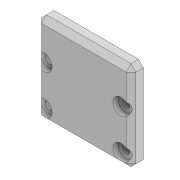
# Autodesk Inventor part: Print_Parts_S2
Saved by Autodesk Inventor 2020.1 (Build 241239000, 239)
## iProperties
Created: 2020-11-09
Part Number: Print_Parts_S2
Material: 一般
Document SubType Name: Modeling
Designer: kenta iguchi
Density: 1 g/cm^3
Appearance: 既定
Author: kenta iguchi
Autodesk Inventor part; units mm, degrees
ref_plane "YZ Plane" through (0, 0, 0) normal (1, 0, 0) x (0, 1, 0)
ref_plane "XZ Plane" through (0, 0, 0) normal (0, 1, 0) x (-1, 0, 0)
ref_plane "XY Plane" through (0, 0, 0) normal (0, 0, 1) x (1, 0, 0)
sketch "スケッチ1" plane through (0, 0, 0) normal (0, 0, 1) x (1, 0, 0)
  line L0 (-19, -18) -> (19, -18)
  line L1 (19, -18) -> (19, 18)
  line L2 (19, 18) -> (-19, 18)
  line L3 (-19, 18) -> (-19, -18)
  line L4 (-19, -18) -> (19, 18) construction
  line L5 (19, -18) -> (-19, 18) construction
  point P0 (0, 0)
  dimension "d0" = 38
  dimension "d1" = 36
  constraints: 12 end point, 2 midpoint, 2 parallel, 1 horizontal, 1 perpendicular
  measures "d0" distance of L2.end L1.end
  measures "d1" distance of L1.end L0.end
extrude "押し出し1" add sketch "スケッチ1" along normal blind 5
chamfer "面取り1" distance 2 angle 45 8 edges at (0, 18, 5) (19, 0, 5) (0, -18, 5) (-19, 0, 5) (19, -18, 2.5) (-19, -18, 2.5) (-19, 18, 2.5) (19, 18, 2.5)
sketch "スケッチ2" plane through (0, 0, 5) normal (0, 0, 1) x (1, 0, 0)
  line L0 (-19, -18) -> (19, -18) projected
  line L1 (19, -18) -> (19, 18) projected
  line L2 (-16, -13) -> (15, -13)
  line L3 (15, -13) -> (15, 3)
  line L4 (15, 3) -> (-16, 3)
  line L5 (-16, 3) -> (-16, -13)
  line L6 (-16, -13) -> (15, 3) construction
  line L7 (15, -13) -> (-16, 3) construction
  point P0 (0, 0)
  point P1 (-0.5, -5)
  dimension "d4" = 31
  dimension "d5" = 16
  dimension "d6" = 5
  dimension "d7" = 4
  constraints: 12 end point, 2 midpoint, 2 parallel, 1 horizontal, 1 perpendicular
  measures "d4" distance of L4.end L3.end
  measures "d5" distance of L3.end L2.end
  measures "d6" distance between parallel lines of L2 L0
  measures "d7" distance between parallel lines of L3 L1
hole "穴1" at (-16, 3, 5) at (-16, -13, 5) at (15, -13, 5) at (15, 3, 5) direction (0, 0, -1) diameter 3.2 depth 6 counterbore diameter 6.5 counterbore depth 2
